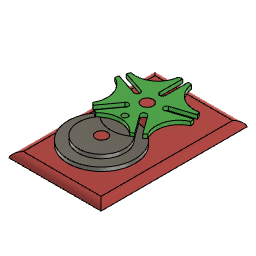
Geneva Wheel Mechanism v4 (Autodesk Fusion 360 design; units mm, degrees)
Autodesk Fusion 360 part; units mm, degrees
note: some values were not read from the file. Set by a fixed rule: which sketch regions a step uses.
sketch "wheel" plane through (0, 0, 0) normal (0, 0, 1) x (1, 0, 0) in component "Wheel"
  line L0 (0, 0) -> (29.389263, -40.45085) construction
  line L1 (0, 0) -> (50, 0) construction
  line L2 (0, 0) -> (-29.389263, -40.45085) construction
  line L3 (0, 0) -> (50, 0) construction
  circle A0 centre (0, -65) radius 38.206041 construction
  line L4 (8.721891, -18.384535) -> (26.355449, -42.655044)
  line L5 (32.423076, -38.246655) -> (14.789519, -13.976145)
  arc A1 (14.789519, -13.976145) -> (8.721891, -18.384535) centre (11.755705, -16.18034) ccw
  line L6 (11.755705, -16.18034) -> (29.389263, -40.45085) construction
  line L7 (20.179944, 2.613878) -> (48.71164, 11.884388)
  arc A2 (17.862317, 9.746802) -> (20.179944, 2.613878) centre (19.02113, 6.18034) ccw
  line L8 (46.394012, 19.017312) -> (17.862317, 9.746802)
  line L9 (3.75, 20) -> (3.75, 50)
  arc A3 (-3.75, 20) -> (3.75, 20) centre (0, 20) ccw
  line L10 (-3.75, 50) -> (-3.75, 20)
  line L11 (-17.862317, 9.746802) -> (-46.394012, 19.017312)
  arc A4 (-20.179944, 2.613878) -> (-17.862317, 9.746802) centre (-19.02113, 6.18034) ccw
  line L12 (-48.71164, 11.884388) -> (-20.179944, 2.613878)
  line L13 (-14.789519, -13.976145) -> (-32.423076, -38.246655)
  arc A5 (-8.721891, -18.384535) -> (-14.789519, -13.976145) centre (-11.755705, -16.18034) ccw
  line L14 (-26.355449, -42.655044) -> (-8.721891, -18.384535)
  circle A6 centre (0, 0) radius 7.5
  arc A7 (22.187174, -44.807692) -> (-22.187174, -44.807692) centre (0, -65) ccw
  arc A8 (-26.272675, -42.541116) -> (-22.187174, -44.807692) centre (0, 0) ccw
  arc A9 (-29.389263, -40.45085) -> (-29.318323, -40.502295) centre (0, 0) ccw
  arc A10 (22.187174, -44.807692) -> (26.272675, -42.541116) centre (0, 0) ccw
  arc A11 (29.318323, -40.502295) -> (29.389263, -40.45085) centre (0, 0) ccw
  arc A12 (49.470862, 7.254918) -> (35.758434, -34.947595) centre (61.818674, -20.086105) ccw
  arc A13 (8.3875, 49.291478) -> (44.287102, 23.208891) centre (38.206041, 52.586105) ccw
  arc A14 (-44.287102, 23.208891) -> (-8.3875, 49.291478) centre (-38.206041, 52.586105) ccw
  arc A15 (-35.758434, -34.947595) -> (-49.470862, 7.254918) centre (-61.818674, -20.086105) ccw
  arc A16 (46.260081, 18.973795) -> (44.287102, 23.208891) centre (0, 0) ccw
  arc A17 (8.3875, 49.291478) -> (3.75, 49.859177) centre (0, 0) ccw
  arc A18 (-3.75, 49.859177) -> (-8.3875, 49.291478) centre (0, 0) ccw
  arc A19 (-44.287102, 23.208891) -> (-46.260081, 18.973795) centre (0, 0) ccw
  arc A20 (32.340302, -38.132727) -> (35.758434, -34.947595) centre (0, 0) ccw
  arc A21 (50, 0) -> (48.577709, 11.840871) centre (0, 0) ccw
  arc A22 (-48.577709, 11.840871) -> (-49.470862, 7.254918) centre (0, 0) ccw
  arc A23 (-35.758434, -34.947595) -> (-32.340302, -38.132727) centre (0, 0) ccw
  dimension "d1" = 100
  dimension "d2" = 50
  dimension "d3" = 54
  dimension "d4" = 126
  dimension "d5" = 50
  dimension "d6" = 65
  dimension "d7" = 60
  dimension "d9" = 20
  dimension "d12" = 15
  dimension "d14" = 360
  constraint coincident L0.start L1.start
  constraint horizontal L1
  constraint horizontal L3
  constraint tangent L0 A0
  constraint tangent L2 A0
  constraint concentric A0 A7
  constraint parallel L4 L5
  constraint tangent L5 A1
  constraint tangent L4 A1
  constraint parallel L0 L6
  constraint concentric A6 A10
  constraint concentric A8 A10
  constraint concentric A9 A10
  constraint concentric A10 A11
  constraint concentric A11 A20
  constraint concentric A16 A20
  constraint concentric A16 A18
  constraint concentric A18 A22
  constraint concentric A16 A17
  constraint concentric A18 A19
  constraint concentric A20 A21
  constraint concentric A22 A23
  measures "d1" diameter of A10
  measures "d3" angle of L0 L1
  measures "d4" angle of L2 L3
  measures "d6" distance of L0.start A0.centre
  measures "d7" diameter of A7
  measures "d12" diameter of A6
extrude "Extrude1" add sketch "wheel" along normal blind 5 makes body 1 in component "Wheel"
sketch "driver" plane through (0, 0, 0) normal (0, 0, 1) x (1, 0, 0) in component "Driver"
  circle A0 centre (7.181347, -66.560205) radius 38.25
  circle A1 centre (7.181347, -66.560205) radius 30
  circle A2 centre (7.181347, -66.560205) radius 32.5
  circle A3 centre (7.181347, -66.560205) radius 7.5
  circle A4 centre (0, -28.990393) radius 3.75
  line L0 (-20.763278, -49.966595) -> (-3.194351, -20.379476)
  line L1 (4.542773, -19.301843) -> (29.528022, -42.961982)
  arc A5 (4.542773, -19.301843) -> (-3.194351, -20.379476) centre (1.104823, -22.932339) ccw
  arc A6 (-15.179332, -46.560205) -> (29.542027, -46.560205) centre (7.181347, -19.634381) ccw
  circle A7 centre (7.181347, -66.560205) radius 43.318279
  point P0 (0, -15)
  dimension "d17" = 76.5
  dimension "d18" = 60
  dimension "d19" = 65
  dimension "d20" = 15
  dimension "d21" = 7.5
  dimension "d22" = 15
  dimension "d23" = 5
  dimension "d24" = 20
  dimension "d25" = 35
  constraint concentric A0 A1
  constraint concentric A1 A2
  constraint concentric A2 A3
  constraint tangent A2 L1
  constraint tangent A2 L0
  constraint coincident P0 L0
  constraint coincident P0 L1
  constraint tangent L0 A5
  constraint tangent L1 A5
  constraint concentric A3 A7
  measures "d17" diameter of A0
  measures "d18" diameter of A1
  measures "d19" diameter of A2
  measures "d20" diameter of A3
  measures "d21" diameter of A4
  measures "d22" distance of P0 origin
  measures "d23" radius of A5
  measures "d25" radius of A6
sketch "suport of the wheel and driver" plane through (0, 0, 0) normal (0, 0, 1) x (1, 0, 0) in component "Table"
  circle A0 centre (0, 0) radius 7.5
  circle A1 centre (7.179062, -66.562709) radius 7.5
  dimension "d30" = 15
  dimension "d35" = 15
  constraint coincident A0.centre origin
  measures "d30" diameter of A0
  measures "d35" diameter of A1
extrude "Extrude1'" add sketch "suport of the wheel and driver" along normal blind -20 and the other way blind -5 separate body contours A0 picked at (1.915775, 2.809925) makes body 2 in component "Table"
extrude "Extrude2" add sketch "driver" along normal blind -20 and the other way blind -5 separate body contours A3 picked at (7.73765, -68.997525) makes body 3 in component "Table"
sketch "table" plane through (0, 0, -20) normal (0, 0, -1) x (1, 0, 0) in component "Table"
  circle A0 centre (7.181347, 66.560205) radius 7.5
  line L0 (60, 120) -> (-60, 120)
  line L1 (-60, 120) -> (-60, -70)
  line L2 (-60, -70) -> (60, -70)
  line L3 (60, -70) -> (60, 120)
  circle A1 centre (7.181347, 66.560205) radius 7.5
  circle A2 centre (0, 0) radius 7.5
  dimension "d42" = 15
  constraint horizontal L0
  constraint vertical L1
  constraint horizontal L2
  constraint vertical L3
  constraint concentric A0 A1
  constraint coincident A2.centre origin
  measures "d42" diameter of A2
extrude "Extrude3" add sketch "table" along normal blind 7 contours A0 A1 | L0 L1 L2 L3 | A2 picked at (6.982095, 68.887389) picked at (0.186825, -49.159676) picked at (1.83263, 1.700432) bodies 2 3 in component "Table"
extrude "Extrude4" cut sketch "table" along normal blind 4 contours A0 A1 | A2 picked at (6.982095, 68.887389) picked at (1.83263, 1.700432) bodies 2 in component "Table"
extrude "Extrude5" add sketch "suport of the wheel and driver" against normal blind 25 bodies 2 in component "Table"
extrude "Extrude3'" add sketch "driver" against normal blind 5 separate body contours A0 A2 L0 L1 | A0 L0 L1 A7 | A0 A2 A4 L0 L1 | A0 A4 L0 L1 A7 | A0 A4 | A0 A4 | A2 | A1 A6 | A1 A6 | A3 picked at (-23.400726, -47.082709) picked at (-13.325267, -30.436111) picked at (-4.866642, -34.386299) picked at (6.629914, -24.987484) picked at (0.1509, -30.244944) picked at (-0.232126, -27.776006) picked at (31.421539, -47.59345) picked at (-9.522362, -58.061132) picked at (4.172239, -48.595854) picked at (7.73765, -68.997525) makes body 4 in component "Driver"
extrude "Extrude4'" add sketch "driver" along normal blind 5 contours A0 A4 | A0 A4 | A1 A6 picked at (0.1509, -30.244944) picked at (-0.232126, -27.776006) picked at (-9.522362, -58.061132) bodies 4 in component "Driver"
fillet "Fillet1" radius 10 4 edges at (60, -25, -20) (0, -120, -20) (-60, -25, -20) (0, 70, -20) on bodies 2 in component "Table"
component "Wheel" placed x (1, 0, 0) y (0, 1, 0) z (0, 0, 1) at (0, 0, 0)
component "Driver" placed x (1, 0, 0) y (0, 1, 0) z (0, 0, 1) at (0, 0, 0)
component "Table" placed x (1, 0, 0) y (0, 1, 0) z (0, 0, 1) at (0, 0, 0)
named bodies: "wheel", "table", "driver"
